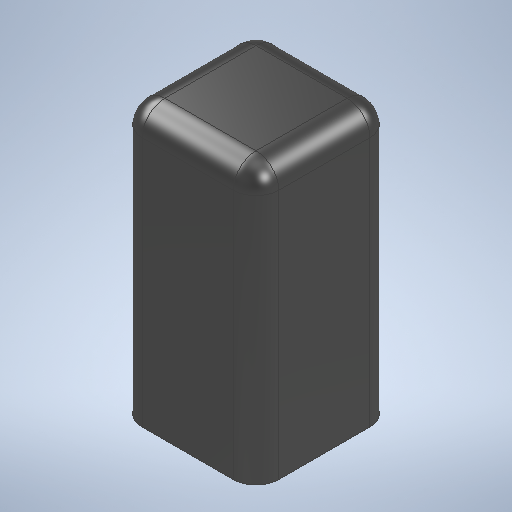
# Autodesk Inventor part: Button
Saved by Autodesk Inventor 2025.3 (Build 293356000, 356)
## iProperties
Created: 2025-05-30
Part Number: Button
Material: Generic
Document SubType Name: Modeling
Designer: delh
Mass: 0.373808 g
Surface Area: 3.80116 cm^2
Volume: 0.373808 cm^3
Density: 1 g/cm^3
Appearance: Default
Author: delh
Autodesk Inventor part; units mm, degrees
ref_plane "YZ Plane" through (0, 0, 0) normal (1, 0, 0) x (0, 1, 0)
ref_plane "XZ Plane" through (0, 0, 0) normal (0, 1, 0) x (-1, 0, 0)
ref_plane "XY Plane" through (0, 0, 0) normal (0, 0, 1) x (1, 0, 0)
sketch "Sketch1" plane through (0, 0, 0) normal (0, 1, 0) x (-1, 0, 0)
  line L0 (3, 3) -> (-3, 3)
  line L1 (-3, 3) -> (-3, -3)
  line L2 (-3, -3) -> (3, -3)
  line L3 (3, -3) -> (3, 3)
  line L4 (3, 3) -> (-3, -3) construction
  line L5 (-3, 3) -> (3, -3) construction
  point P0 (0, 0)
  dimension "d0" = 6
  dimension "d1" = 6
  constraints: 12 end point, 2 midpoint, 2 parallel, 1 horizontal, 1 perpendicular
  measures "d0" distance of L2.end L1.end
  measures "d1" distance of L1.end L0.end
extrude "Extrusion1" add sketch "Sketch1" along normal blind 12
sketch "Sketch2" plane through (0, 0, 0) normal (0, -1, 0) x (1, 0, 0)
  line L0 (-1.7, -1.7) -> (1.7, -1.7)
  line L1 (1.7, -1.7) -> (1.7, 1.7)
  line L2 (1.7, 1.7) -> (-1.7, 1.7)
  line L3 (-1.7, 1.7) -> (-1.7, -1.7)
  line L4 (-1.7, -1.7) -> (1.7, 1.7) construction
  line L5 (1.7, -1.7) -> (-1.7, 1.7) construction
  point P0 (0, 0)
  dimension "d4" = 3.4
  dimension "d5" = 3.4
  constraints: 12 end point, 2 midpoint, 2 parallel, 1 horizontal, 1 perpendicular
  measures "d4" distance of L2.end L1.end
  measures "d5" distance of L1.end L0.end
extrude "Extrusion2" cut sketch "Sketch2" against normal blind 3.8
sketch "Sketch3" plane through (0, 0, 0) normal (0, 0, 1) x (1, 0, 0)
  line L0 (-1.65, 0.7481) -> (1.65, 0.7481) projected
  line L1 (1.25, 1.7481) -> (1.25, 0.7481) projected
  line L2 (-1.65, 1.7481) -> (1.65, 1.7481) projected
  line L3 (-1.25, 0.7481) -> (-1.25, 1.7481) projected
  line L4 (1.7, 0) -> (1.7, 3.8) projected
  line L5 (1.7, 1.6241) -> (1.6, 1.6241)
  line L6 (1.6, 1.6241) -> (1.6, 0.8418)
  line L7 (1.6, 0.8418) -> (1.7, 0.8418)
  line L8 (1.7, 0.8418) -> (1.7, 1.6241)
  point P0 (0, 0)
  dimension "d8" = 0.1
  constraints: 8 end point, 2 parallel, 1 horizontal, 1 perpendicular, 1 point on line
  measures "d8" distance between parallel lines of L6 L4
extrude "Extrusion3" add sketch "Sketch3" along normal mid plane 3.8 contours L7 L6 L5 L4
mirror "Mirror1" about plane through (0, 0, 0) normal (1, 0, 0) of "Extrusion3"
fillet "Fillet1" radius 0.1 2 edges at (-1.6, 0.8418, 0) (1.6, 0.8418, 0)
fillet "Fillet2" radius 1 8 edges at (-3, 6, 3) (3, 6, 3) (3, 6, -3) (-3, 6, -3) (0, 12, 3) (-3, 12, 0) (0, 12, -3) (3, 12, 0)
body "Solid1"
